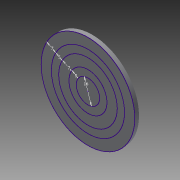
# Autodesk Inventor part: Marker1
Saved by Autodesk Inventor 2014 SP1 (Build 180222100, 222)
## iProperties
Created: 2014-07-16
Part Number: Marker1
Material: Generic
Document SubType Name: Modeling
Designer: Erin
Density: 1 g/cm^3
Appearance: Default
Author: Erin
Autodesk Inventor part; units mm, degrees
ref_plane "YZ Plane" through (0, 0, 0) normal (1, 0, 0) x (0, 1, 0)
ref_plane "XZ Plane" through (0, 0, 0) normal (0, 1, 0) x (-1, 0, 0)
ref_plane "XY Plane" through (0, 0, 0) normal (0, 0, 1) x (1, 0, 0)
sketch "Sketch1" plane through (0, 0, 0) normal (0, 1, 0) x (-1, 0, 0)
  circle A0 centre (0, 0) radius 8
  circle A1 centre (0, 0) radius 13
  circle A2 centre (0, 0) radius 20
  circle A3 centre (0, 0) radius 25
  circle A4 centre (0, 0) radius 32
  dimension "d0" = 16
  dimension "d1" = 5
  dimension "d2" = 7
  dimension "d3" = 5
  dimension "d4" = 7
  constraints: 5 centre point, 5 coincident
  measures "d0" diameter of A0
  measures "d1" radial gap between concentric circles of A1 A0
  measures "d2" radial gap between concentric circles of A2 A1
  measures "d3" radial gap between concentric circles of A3 A2
  measures "d4" radial gap between concentric circles of A4 A3
extrude "Extrusion1" add sketch "Sketch1" along normal blind 1.5 contours A0 | A1 | A2 | A3 | A4
extrude "Extrusion2" add sketch "Sketch1" along normal blind 3
body "Solid1"
